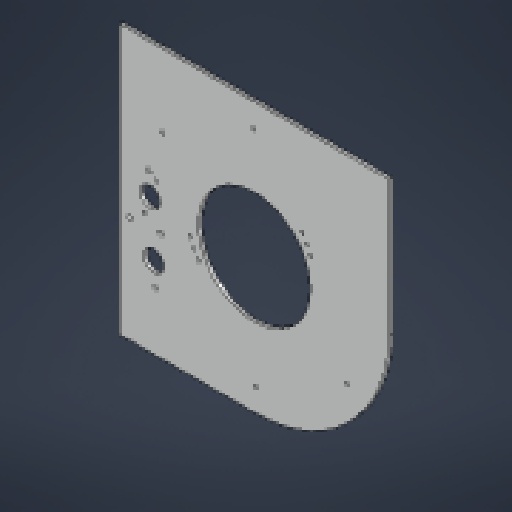
# Autodesk Inventor part: PLATE,SHOOTER,MOUNT
Saved by Autodesk Inventor 2026 (Build 300175000, 175)
## iProperties
Created: 2026-02-09
Part Number: PLATE,SHOOTER,MOUNT
Material: Aluminum 6061
Document SubType Name: Sheet Metal
Designer: littl
Density: 2.7 g/cm^3
Sheet Metal Rule: Default
Appearance: Aluminum - Flat
Mass: 1327.53 g
Surface Area: 2156.48 cm^2
Volume: 491.678 cm^3
Author: littl
Autodesk Inventor part; units mm, degrees
ref_plane "YZ Plane" through (0, 0, 0) normal (1, 0, 0) x (0, 1, 0)
ref_plane "XZ Plane" through (0, 0, 0) normal (0, 1, 0) x (-1, 0, 0)
ref_plane "XY Plane" through (0, 0, 0) normal (0, 0, 1) x (1, 0, 0)
sketch "Sketch1" plane through (0, 0, 0) normal (0, 0, 1) x (1, 0, 0)
  line L0 (-190.5, -190.5) -> (190.5, -190.5)
  line L1 (190.5, -190.5) -> (190.5, 190.5)
  line L2 (190.5, 190.5) -> (-190.5, 190.5)
  line L3 (-190.5, 190.5) -> (-190.5, -190.5)
  line L4 (-190.5, -190.5) -> (190.5, 190.5) construction
  line L5 (190.5, -190.5) -> (-190.5, 190.5) construction
  circle A0 centre (0, 0) radius 79.375
  line L6 (130.599, -90.0738) -> (-0.5713, 156.6217) construction
  line L7 (-0.5713, 156.6217) -> (-129.5258, 88.0554) construction
  line L8 (-129.5258, 88.0554) -> (1.6445, -158.6401) construction
  line L9 (1.6445, -158.6401) -> (130.599, -90.0738) construction
  line L10 (130.599, -90.0738) -> (-129.5258, 88.0554) construction
  line L11 (-0.5713, 156.6217) -> (1.6445, -158.6401) construction
  line L12 (1.6445, -158.6401) -> (-64.4772, -34.2832) construction
  line L13 (-64.4772, -34.2832) -> (-12.5828, -6.6904) construction
  line L14 (-65.0486, 122.3386) -> (66.1218, -124.357) construction
  line L15 (-91.2837, -21.0636) -> (-75.8652, -12.8655) construction
  line L16 (-91.2837, -21.0636) -> (-85.3214, -32.2771) construction
  line L17 (-85.3214, -32.2771) -> (-79.3591, -43.4905) construction
  line L18 (68.5077, 63.899) -> (53.0893, 55.7008) construction
  line L19 (68.5077, 63.899) -> (74.47, 52.6855) construction
  line L20 (74.47, 52.6855) -> (80.4323, 41.4721) construction
  arc A1 (0, -190.5) -> (190.5, 0) centre (0, 0) ccw
  point P0 (0.5366, -1.0092)
  point P1 (152.4, 190.5)
  point P2 (-17.6976, -190.5)
  dimension "d0" = 381
  dimension "d1" = 158.75
  dimension "d2" = 279.4
  dimension "d3" = 146.05
  dimension "d4" = 28
  dimension "d5" = 140.843
  dimension "d6" = 114.3
  dimension "d7" = 17.4625
  dimension "d8" = 12.7
  dimension "d9" = 114.3
  dimension "d11" = 17.4625
  dimension "d12" = 12.7
  constraints: 42 end point, 8 midpoint, 7 point on line, 6 coincident, 6 parallel, 5 perpendicular, 3 equal length, 2 centre point, 2 collinear, 2 point on circle, 1 horizontal
  measures "d0" distance of L2.end L1.end
  measures "d1" diameter of A0
  measures "d2" distance of L6.start L6.end
  measures "d3" distance of L6.end L7.end
  measures "d4" angle of L3 L8
  measures "d5" distance of L8.end L12.end
  measures "d6" distance between parallel lines of L7 L15
  measures "d7" distance of L15.start L15.end
  measures "d8" distance of L15.start L16.end
  measures "d9" distance between parallel lines of L7 L18
  measures "d11" distance of L18.start L18.end
  measures "d12" distance of L19.end L20.end
extrude "Plate1" add sketch "Sketch1" along normal blind 4.7752 contours L3 L2 L1 A1 L0
hole "Hole1" at (-129.5258, 88.0554, 0) at (1.6445, -158.6401, 0) at (-0.5713, 156.6217, 0) at (130.599, -90.0738, 0) at (-91.2837, -21.0636, 0) at (-85.3214, -32.2771, 0) at (-79.3591, -43.4905, 0) at (68.5077, 63.899, 0) at (74.47, 52.6855, 0) at (80.4323, 41.4721, 0) direction (0, 0, 1) diameter 4.9784 end through all clearance for "Flat Head Machine Screw (82)" size "#10" standard "Ansi Unified Screw Threads"
sketch "Sketch2" plane through (0, 0, 4.7752) normal (0, 0, 1) x (1, 0, 0)
  circle A0 centre (-147.32, 0) radius 15.5575 construction
  circle A1 centre (-142.2455, -76.0308) radius 15.5575 construction
  line L0 (-147.32, 0) -> (0, 0) construction
  line L1 (0, 0) -> (-142.2455, -76.0308) construction
  circle A2 centre (-142.2455, -76.0308) radius 40.64
  circle A3 centre (-147.32, 0) radius 26.67
  point P0 (-130.6842, -94.531)
  dimension "d23" = 147.32
  dimension "d24" = 31.115
  dimension "d26" = 161.29
  dimension "d35" = 161.29
  dimension "d36" = 81.28
  dimension "d37" = 53.34
  dimension "d76" = 76.2
  constraints: 4 centre point, 4 coincident, 4 end point, 1 equal radius, 1 horizontal
  measures "d23" distance of point (-147.32, 0) L0.end
  measures "d24" diameter of A0
  measures "d26" distance of L0.end point (-142.245, -76.031)
  measures "d35" distance of L0.end point (-130.684, -94.531)
  measures "d36" diameter of A2
  measures "d37" diameter of A3
  measures "d76" distance of point (-142.245, -76.031) L0.start
hole "Hole2" at (-147.32, 0, 4.7752) at (-142.2455, -76.0308, 4.7752) direction (0, 0, -1) diameter 28.575 end through all
sketch "Sketch3" plane through (0, 0, 4.7752) normal (0, 0, 1) x (1, 0, 0)
  circle A0 centre (-147.32, 0) radius 14.2875 construction
  circle A1 centre (-142.2455, -76.0308) radius 14.2875 construction
  line L0 (-147.32, 0) -> (-142.2455, -76.0308) construction
  line L1 (-147.32, 0) -> (-149.4344, 31.6795) construction
  line L2 (-142.2455, -76.0308) -> (-139.7082, -114.0463) construction
  line L3 (-132.1109, -37.1697) -> (-144.7827, -38.0154) construction
  line L4 (-176.4623, -40.1298) -> (-144.7827, -38.0154) construction
  point P0 (0, 0)
  dimension "d77" = 31.75
  dimension "d78" = 38.1
  dimension "d79" = 12.7
  dimension "d80" = 31.75
  constraints: 10 end point, 2 collinear, 2 midpoint, 2 perpendicular
  measures "d77" distance of L0.start L1.end
  measures "d78" distance of L0.end L2.end
  measures "d79" distance of L3.start L3.end
  measures "d80" distance of L4.start L3.end
hole "Hole3" at (-132.1109, -37.1697, 4.7752) at (-176.4623, -40.1298, 4.7752) at (-139.7082, -114.0463, 4.7752) at (-149.4344, 31.6795, 4.7752) direction (0, 0, -1) diameter 6.5278 end through all clearance for "Flat Head Machine Screw (82)" size "1/4" standard "Ansi Unified Screw Threads"
sketch "Sketch5" plane through (0, 0, 4.7752) normal (0, 0, 1) x (1, 0, 0)
  circle A0 centre (-147.32, 0) radius 14.2875 construction
  line L0 (-160.02, 21.997) -> (-147.32, 0) construction
  line L1 (-147.32, 0) -> (-147.32, 17.1692) construction
  circle A1 centre (-142.2455, -76.0308) radius 14.2875 projected
  line L2 (-142.2455, -76.0308) -> (-125.9187, -56.5733) construction
  point P0 (0, 0)
  point P1 (-134.62, -21.997)
  point P2 (-158.5723, -95.4884)
  dimension "d63" = 25.4
  dimension "d66" = 360
  dimension "d84" = 360
  dimension "d86" = 40
  dimension "d87" = 30
  constraints: 6 end point, 1 coincident, 1 equal length, 1 vertical, 6 other
  measures "d63" distance of L0.start L0.end
  measures "d86" angle of L1 L2
  measures "d87" angle of L1 L0
hole "Hole5" at (-160.02, 21.997, 4.7752) at (-134.62, -21.997, 4.7752) at (-158.5723, -95.4884, 4.7752) at (-125.9187, -56.5733, 4.7752) direction (0, 0, -1) diameter 4.9784 end through all clearance for "Flat Head Machine Screw (82)" size "#10" standard "Ansi Unified Screw Threads"
equation "\"d11\" = d7"
equation "\"d19\" = Thickness"
equation "\"d35\" = d26"
equation "\"d52\" = Thickness"
equation "\"d13\" = Thickness"
equation "\"BendRadius\" = Thickness"
equation "\"BendReliefWidth\" = Thickness"
equation "\"BendReliefDepth\" = 0.5 * Thickness"
equation "\"CornerReliefSize\" = 4 * Thickness"
equation "\"MinimumRemnant\" = 2 * Thickness"
equation "\"TransitionRadius\" = BendRadius"
equation "\"JacobiRadiusSize\" = BendRadius"
equation "\"GapSize\" = Thickness"
equation "\"Thickness\" = 4.7752"
body "Solid1"
